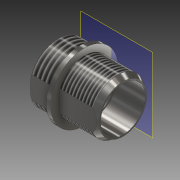
# Autodesk Inventor part: корпус разъема
Saved by Autodesk Inventor 2018.1 (Build 221171000, 171)
## iProperties
Created: 2019-07-16
Part Number: корпус разъема
Material: Сталь, нержавеющая, полированная
Document SubType Name: Modeling
Designer: Boss
Mass: 5.34784 g
Surface Area: 12.0029 cm^2
Volume: 0.66848 cm^3
Density: 8 g/cm^3
Appearance: Нержавеющая — полированная
inside: 10,000 мм
Author: Boss
Autodesk Inventor part; units mm, degrees
ref_plane "YZ Plane" through (0, 0, 0) normal (1, 0, 0) x (0, 1, 0)
ref_plane "XY Plane" through (0, 0, 0) normal (0, 0, 1) x (1, 0, 0)
sketch "Эскиз1" plane through (0, 0, 0) normal (0, 0, 1) x (1, 0, 0)
  line L0 (-7.8, 4.75) -> (0, 4.75)
  line L1 (0, 4.75) -> (0, 5)
  line L2 (0, 5) -> (6.5, 5)
  line L3 (6.5, 5) -> (6.5, 5.3)
  line L4 (6.5, 5.3) -> (5.2876, 6)
  line L5 (5.2876, 6) -> (-2.1, 6)
  line L6 (-2.1, 6) -> (-2.1, 7.5)
  line L7 (-2.1, 7.5) -> (-3.1, 7.5)
  line L8 (-3.1, 7.5) -> (-3.1, 6.5)
  line L9 (-3.1, 6.5) -> (-7.8, 6.5)
  line L10 (-6.6244, 0) -> (6.6244, 0) construction
  line L11 (-8.1, 6.2) -> (-8.1, 5.05)
  line L12 (-7.8, 6.5) -> (-8.1, 6.2)
  line L13 (-8.1, 5.05) -> (-7.8, 4.75)
  point P0 (0, 0)
  point P1 (-8.1, 6.5)
  point P2 (-8.1, 4.75)
  point P3 (0, 0)
  dimension "d2" = 12
  dimension "d3" = 15
  dimension "d8" = 13
  dimension "d9" = 1
  dimension "d10" = 0.3
  dimension "d11" = 120
  dimension "d12" = 6.5
  dimension "d14" = 0.3
  dimension "d15" = 0.3
  dimension "d16" = 0.3
  dimension "d17" = 0.3
  dimension "d18" = 9.5
  dimension "d19" = 5
  dimension "d20" = 1
  dimension "d21" = 8.6
  dimension "inside" = 10
  constraints: 28 end point, 4 point on line, 2 perpendicular, 1 coincident, 1 horizontal, 1 midpoint, 1 parallel, 1 vertical alignment
  measures "d2" diameter of L5 L10
  measures "d3" diameter of L7 L10
  measures "d8" diameter of L9 L10
  measures "d9" distance between parallel lines of L5 L2
  measures "d10" distance of L2.end L3.end
  measures "d11" angle of L4 L3
  measures "d12" distance between parallel lines of L3 L1
  measures "d14" distance of L9.end point (-8.1, 6.5)
  measures "d15" distance of L11.start point (-8.1, 6.5)
  measures "d16" distance of L11.end point (-8.1, 4.75)
  measures "d17" distance of L0.start point (-8.1, 4.75)
  measures "d18" diameter of L0 L10
  measures "d19" distance between parallel lines of L11 L8
  measures "d20" distance between parallel lines of L6 L8
  measures "d21" distance between parallel lines of L6 L3
  measures "inside" diameter of L2 L10
revolve "Вращение1" add sketch "Эскиз1" angle 360 about axis through (-6.6244, 0, 0) along (1, 0, 0)
thread "Резьба1" size "M14x1" class "6g" standard "ANSI Metric M Profile" full length
thread "Резьба2" size "M12x0.75" class "6g" standard "ANSI Metric M Profile" full length
ref_plane "РабПлоскость1" through (1.5938, 6, 0) normal (0, 1, 0) x (-1, 0, 0)
sketch "Эскиз2" plane through (1.5938, 6, 0) normal (0, 1, 0) x (-1, 0, 0)
  line L0 (3.6938, 5) -> (-6.3062, 5)
  line L1 (-6.3062, 5) -> (-6.3062, -5)
  line L2 (-6.3062, -5) -> (3.6938, -5)
  line L3 (3.6938, -5) -> (3.6938, 5)
  line L4 (3.6938, 7.5) -> (3.6938, -7.5) projected
  point P0 (1.5938, 0)
  point P1 (-6.3062, 0)
  point P2 (3.6938, 0)
  dimension "d28" = 10
  dimension "d29" = 10
  constraints: 8 end point, 2 horizontal alignment, 2 midpoint, 1 collinear
  measures "d28" distance between parallel lines of L2 L0
  measures "d29" distance between parallel lines of L1 L3
extrude "Выдавливание1" cut sketch "Эскиз2" against normal blind 0.5
sketch "Эскиз3" plane through (1.5938, 6, 0) normal (0, 1, 0) x (-1, 0, 0)
  line L0 (4.6938, 7.5) -> (4.6938, -7.5) projected
  line L1 (4.6938, -4) -> (12.6938, -4)
  line L2 (12.6938, -4) -> (12.6938, 4)
  line L3 (12.6938, 4) -> (4.6938, 4)
  line L4 (4.6938, 4) -> (4.6938, -4)
  point P0 (1.5938, 0)
  point P1 (4.6938, 0)
  dimension "d32" = 8
  dimension "d33" = 8
  constraints: 8 end point, 1 collinear, 1 horizontal alignment, 1 midpoint
  measures "d32" distance of L3.end L2.end
  measures "d33" distance of L2.end L1.end
extrude "Выдавливание2" cut sketch "Эскиз3" along normal blind 0.5
mirror "Зеркальное отражение1" about plane through (0, 0, 0) normal (0, 1, 0) of "Выдавливание1", "Выдавливание2"
equation "\"d15\" = d14"
equation "\"d16\" = d14"
equation "\"d17\" = d16"
equation "\"d29\" = d28"
